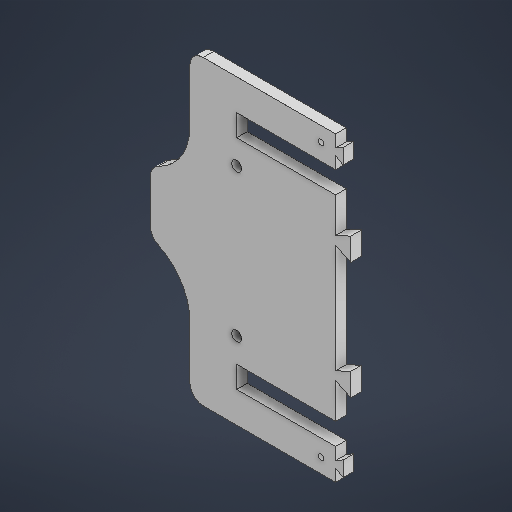
# Autodesk Inventor part: platform_deck_v3_3
Saved by Autodesk Inventor 2026.1 (Build 301233020, 233B)
## iProperties
Created: 2026-01-28
Part Number: platform_deck_v3_3
Material: Genérico
Document SubType Name: Modeling
Designer: i5
Density: 1 g/cm^3
Appearance: Valor por defecto
Author: i5
Autodesk Inventor part; units mm, degrees
ref_plane "YZ Plane" through (0, 0, 0) normal (1, 0, 0) x (0, 1, 0)
ref_plane "XZ Plane" through (0, 0, 0) normal (0, 1, 0) x (-1, 0, 0)
ref_plane "XY Plane" through (0, 0, 0) normal (0, 0, 1) x (1, 0, 0)
sketch "Boceto1" plane through (0, 0, 0) normal (0, 0, 1) x (1, 0, 0)
  line L0 (110.3805, 180) -> (110.3805, 172.7)
  line L1 (110.3805, 161.5) -> (110.3805, 168.8)
  line L2 (114.9005, 170.75) -> (114.9005, 175.3)
  line L3 (114.9005, 175.3) -> (110.3805, 172.7)
  line L4 (114.9005, 170.75) -> (114.9005, 166.2)
  line L5 (114.9005, 166.2) -> (110.3805, 168.8)
  line L6 (110.3805, 148.5) -> (110.3805, 127.5)
  line L7 (119.4805, 124.95) -> (119.4805, 131.75)
  line L8 (119.4805, 131.75) -> (110.3805, 127.5)
  line L9 (119.4805, 124.95) -> (119.4805, 118.15)
  line L10 (119.4805, 118.15) -> (110.3805, 122.4)
  line L11 (110.3805, 122.4) -> (110.3805, 90)
  line L12 (110.3805, 161.5) -> (51.3805, 161.5)
  line L13 (110.3805, 148.5) -> (51.3805, 148.5)
  line L14 (51.3805, 148.5) -> (51.3805, 161.5)
  line L15 (110.3805, 180) -> (31.3805, 180)
  line L16 (-0.0195, 90) -> (-0.0195, 103.12)
  arc A0 (4.5767, 110.3598) -> (-0.0195, 103.12) centre (7.9805, 103.12) ccw
  arc A1 (31.3805, 180) -> (23.3805, 172) centre (31.3805, 172) ccw
  arc A2 (4.5767, 110.3598) -> (23.3805, 139.9789) centre (-9.3489, 139.9789) ccw
  line L17 (23.3805, 139.9789) -> (23.3805, 172)
  circle A3 centre (101.7305, 171.35) radius 1.65
  circle A4 centre (51.3805, 133.9) radius 3
  line L18 (110.3805, 0) -> (110.3805, 7.3)
  line L19 (110.3805, 18.5) -> (110.3805, 11.2)
  line L20 (114.9005, 9.25) -> (114.9005, 4.7)
  line L21 (114.9005, 4.7) -> (110.3805, 7.3)
  line L22 (114.9005, 9.25) -> (114.9005, 13.8)
  line L23 (114.9005, 13.8) -> (110.3805, 11.2)
  line L24 (110.3805, 31.5) -> (110.3805, 52.5)
  line L25 (119.4805, 55.05) -> (119.4805, 48.25)
  line L26 (119.4805, 48.25) -> (110.3805, 52.5)
  line L27 (119.4805, 55.05) -> (119.4805, 61.85)
  line L28 (119.4805, 61.85) -> (110.3805, 57.6)
  line L29 (110.3805, 57.6) -> (110.3805, 90)
  line L30 (110.3805, 18.5) -> (51.3805, 18.5)
  line L31 (110.3805, 31.5) -> (51.3805, 31.5)
  line L32 (51.3805, 31.5) -> (51.3805, 18.5)
  line L33 (110.3805, 0) -> (31.3805, 0)
  line L34 (-0.0195, 90) -> (-0.0195, 76.88)
  arc A5 (-0.0195, 76.88) -> (4.5767, 69.6402) centre (7.9805, 76.88) ccw
  arc A6 (23.3805, 8) -> (31.3805, 0) centre (31.3805, 8) ccw
  arc A7 (23.3805, 40.0211) -> (4.5767, 69.6402) centre (-9.3489, 40.0211) ccw
  line L35 (23.3805, 40.0211) -> (23.3805, 8)
  circle A8 centre (101.7305, 8.65) radius 1.65
  circle A9 centre (51.3805, 46.1) radius 3
  point P0 (0, 0)
  constraints: 72 end point, 12 point on circle, 10 centre point
extrude "Extrusión1" add sketch "Boceto1" along normal blind 6.35
fillet "Empalme1" radius 0.01 22 edges at (25.7236, 177.6569, 6.35) (23.3805, 155.9894, 6.35) (18.2825, 122.437, 6.35) (1.2266, 107.4077, 6.35) (-0.0195, 96.56, 6.35) (1.2266, 72.5923, 6.35) (18.2825, 57.563, 6.35) (23.3805, 24.0106, 6.35) (25.7236, 2.3431, 6.35) (70.8805, 0, 6.35) (70.8805, 180, 6.35) (25.7236, 177.6569, 0) (23.3805, 155.9894, 0) (18.2825, 122.437, 0) (1.2266, 107.4077, 0) (-0.0195, 96.56, 0) (1.2266, 72.5923, 0) (18.2825, 57.563, 0) (23.3805, 24.0106, 0) (25.7236, 2.3431, 0) (70.8805, 0, 0) (70.8805, 180, 0)
